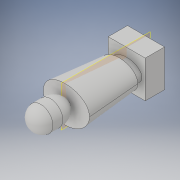
# Autodesk Inventor part: Head Em
Saved by Autodesk Inventor 2017 (Build 210142000, 142)
## iProperties
Created: 2020-02-27
Part Number: Head Em
Material: Generic
Document SubType Name: Modeling
Designer: 10042265
Density: 1 g/cm^3
Appearance: Default
Author: 10042265
Autodesk Inventor part; units mm, degrees
note: some values were not read from the file. Chosen so that the rebuilt part matches the saved one: offset side.
ref_plane "YZ Plane" through (0, 0, 0) normal (1, 0, 0) x (0, 1, 0)
ref_plane "XZ Plane" through (0, 0, 0) normal (0, 1, 0) x (-1, 0, 0)
ref_plane "XY Plane" through (0, 0, 0) normal (0, 0, 1) x (1, 0, 0)
sketch "Sketch1" plane through (0, 0, 0) normal (0, 0, 1) x (1, 0, 0)
  line L0 (0, 0) -> (14.605, 0)
  line L1 (14.605, 0) -> (14.605, 14.605)
  line L2 (14.605, 14.605) -> (0, 14.605)
  line L3 (0, 14.605) -> (0, 0)
  dimension "d0" = 14.605
  dimension "d1" = 14.605
  constraints: 8 end point, 3 perpendicular, 1 horizontal
  measures "d0" distance of L0.start L0.end
  measures "d1" distance of L0.end L1.end
extrude "Extrusion1" add sketch "Sketch1" along normal blind 7.62
sketch "Sketch2" plane through (0, 0, 7.62) normal (0, 0, 1) x (1, 0, 0)
  line L0 (0, 14.605) -> (0, 0) construction
  ellipse E0 centre (7.3072, 7.3024) end of major axis (1.3128, 7.3024) minor radius 3.937
  line L1 (0, 7.3025) -> (14.605, 7.3025) construction
  line L2 (14.605, 0) -> (14.605, 14.605) construction
  line L3 (14.605, 14.605) -> (0, 14.605) construction
  line L4 (7.3025, 14.605) -> (7.3025, 0) construction
  dimension "d4" = 5.9944
  dimension "d5" = 3.937
  constraints: 4 end point, 3 midpoint, 1 vertical, 2 other
extrude "Extrusion2" add sketch "Sketch2" along normal blind 2.921
sketch "Sketch3" plane through (0, 0, 10.541) normal (0, 0, 1) x (1, 0, 0)
  ellipse E0 centre (7.3072, 7.3024) end of major axis (13.3016, 7.3024) minor radius 3.937 projected
  spline S0 degree 5 poles (14.5716, 7.3024) (14.5717, 8.0461) (14.3916, 8.7933) (14.0323, 9.4723) (13.0501, 10.6949) (11.7205, 11.5346) (10.9816, 11.8705) (9.3959, 12.3858) (7.7364, 12.5528) (6.878, 12.5526) (5.2185, 12.3861) (3.6327, 11.8703) (2.8939, 11.535) (1.5642, 10.6942) (0.582, 9.4731) (0.2226, 8.7917) (-0.1371, 7.3024) (0.2226, 5.8131) (0.582, 5.1317) (1.5642, 3.9106) (2.8939, 3.0697) (3.6327, 2.7345) (5.2185, 2.2187) (6.878, 2.0522) (7.7364, 2.052) (9.3959, 2.219) (10.9816, 2.7342) (11.7205, 3.0702) (13.0501, 3.9099) (14.0323, 5.1325) (14.3916, 5.8115) (14.5717, 6.5587) (14.5716, 7.3024) knots 0 0 0 0 0 0 0.094174 0.094174 0.094174 0.196027 0.196027 0.196027 0.303973 0.303973 0.303973 0.405825 0.405825 0.405825 0.5 0.5 0.5 0.594175 0.594175 0.594175 0.696027 0.696027 0.696027 0.803973 0.803973 0.803973 0.905826 0.905826 0.905826 1 1 1 1 1 1
  point P0 (0, 0)
  dimension "d8" = 1.27
  constraints: 1 other
extrude "Extrusion3" add sketch "Sketch3" along normal blind 21.336 draft 5 contours E0 | S0
ref_plane "Work Plane1" through (7.3025, 0, 0) normal (1, 0, 0) x (0, 0, -1)
sketch "Sketch4" plane through (7.3025, 0, 0) normal (1, 0, 0) x (0, 0, -1)
  line L0 (-31.877, 14.376) -> (-31.877, 0.2287) projected
  line L1 (-10.541, 7.3024) -> (-31.877, 7.3024) projected
  line L2 (-10.541, 12.5094) -> (-10.541, 2.0954) projected
  line L3 (-31.877, 14.376) -> (-31.877, 0.2287) projected
  line L4 (-10.541, 7.3024) -> (-31.877, 7.3024) projected
  line L5 (-10.541, 12.5094) -> (-10.541, 2.0954) projected
  arc A0 (-31.877, 0.2287) -> (-31.877, 14.376) centre (-83.9662, 7.3024) ccw
  point P0 (0, 0)
  constraints: 2 point on circle, 1 centre point
extrude "Extrusion4" cut sketch "Sketch4" along normal mid plane 21.336
sketch "Sketch5" plane through (7.3025, 0, 0) normal (1, 0, 0) x (0, 0, -1)
  line L0 (-10.541, 7.3024) -> (-31.3989, 7.3024) projected
  line L1 (-10.541, 7.3024) -> (-31.3989, 7.3024) projected
  line L2 (-10.541, 12.5094) -> (-10.541, 2.0954) projected
  line L3 (-41.5504, 12.175) -> (-37.6803, 12.175)
  arc A0 (-30.6609, 7.3024) -> (-37.6803, 12.175) centre (-37.2928, 5.2409) ccw
  arc A1 (-41.5504, 12.175) -> (-45.7759, 7.3024) centre (-40.8549, 7.3034) ccw
  line L4 (-45.7759, 7.3024) -> (-30.6609, 7.3024)
  point P0 (0, 0)
  constraints: 4 end point, 4 point on circle, 2 centre point, 2 horizontal, 1 vertical alignment, 2 other
revolve "Revolution1" add sketch "Sketch5" angle 360 about axis through (7.3025, 7.3024, 45.7759) along (0, 0, -1)
body "Solid1"
